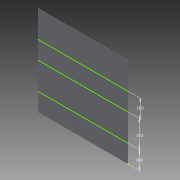
# Autodesk Inventor part: Part17
Saved by Autodesk Inventor 2015 SP2 (Build 190223200, 223)
## iProperties
Created: 2017-05-28
Part Number: Part17
Material: Generic
Document SubType Name: Sheet Metal
Designer: MehariK
Density: 1 g/cm^3
Sheet Metal Rule: Default_mm
Appearance: Default
Author: MehariK
Autodesk Inventor part; units mm, degrees
ref_plane "YZ Plane" through (0, 0, 0) normal (1, 0, 0) x (0, 1, 0)
ref_plane "XZ Plane" through (0, 0, 0) normal (0, 1, 0) x (-1, 0, 0)
ref_plane "XY Plane" through (0, 0, 0) normal (0, 0, 1) x (1, 0, 0)
sketch "Sketch1" plane through (0, 0, 0) normal (0, 1, 0) x (-1, 0, 0)
  line L0 (0, 0) -> (500, 0)
  line L1 (500, 0) -> (500, 500)
  line L2 (500, 500) -> (0, 500)
  line L3 (0, 500) -> (0, 0)
  line L4 (500, 500) -> (0, 500)
  line L5 (0, 0) -> (500, 0)
  dimension "d0" = 500
  dimension "d1" = 500
  constraints: 12 end point, 4 equal length, 1 horizontal, 1 perpendicular
  measures "d0" distance of L2.end L1.end
  measures "d1" distance of L2.end L0.start
sketch "Sketch2" plane through (0, 0, 0) normal (0, 1, 0) x (-1, 0, 0)
  line L0 (500.3847, 350) -> (0, 350)
  line L1 (500.3847, 250) -> (0, 250)
  line L2 (500.3847, 100) -> (0, 100)
  point P0 (0, 0)
  dimension "d3" = 100
  dimension "d4" = 150
  dimension "d5" = 100
  constraints: 6 end point, 3 horizontal
  measures "d3" distance of point (0, 0) L2.end
  measures "d4" distance of L2.end L1.end
  measures "d5" distance of L1.end L0.end
extrude "Plate1" add sketch "Sketch1" along normal blind 0.5
equation "\"BendRadius\" = Thickness"
equation "\"BendReliefWidth\" = Thickness"
equation "\"BendReliefDepth\" = 0.5 * Thickness"
equation "\"CornerReliefSize\" = 4 * Thickness"
equation "\"MinimumRemnant\" = 2 * Thickness"
equation "\"TransitionRadius\" = BendRadius"
equation "\"JacobiRadiusSize\" = BendRadius"
equation "\"GapSize\" = Thickness"
equation "\"d6\" = BendRadius"
equation "\"Thickness\" = 0.5"
body "Solid1"
